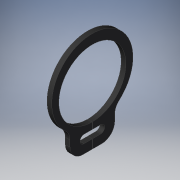
# Autodesk Inventor part: SL-STWS6
Saved by Autodesk Inventor 2019 (Build 230136000, 136)
## iProperties
Created: 2023-09-15
Part Number: SL-STWS6
Material: Generic
Catalog Web Link: www.cadenas.de
Description: SL-STWS, SH-STWS, SHD-STWS-(Precision cleaning) Retaining Rings - External, C-Type
Vendor: MISUMI
Document SubType Name: Modeling
Designer: psAdmin
Manufacturer: MISUMI
Mass: 0.00671227 g
Surface Area: 0.53562 cm^2
Volume: 0.00671227 cm^3
Density: 1 g/cm^3
Appearance: PSOLRGB-175-175-175
Category: PARTsolutions
Company: MISUMI
Title: SL-STWS6
Author: Cadenas PARTsolutions
Comments: (Precision cleaning) Retaining Rings - External, C-Type
PSOL_IDENT_0: {$CADENAS_DATA/23d-libs/misumi/metric/28_keys_magnets/sl_stws.prj},178 {VTYP=3D},{NB=SL-STWS6},{LINA=
PSOL_IDENT_1: SL-STWS6},{NN=SL-STWS, SH-STWS, SHD-STWS},{DATE=01.06.2023 05:14:51},{GEOMDATE=23.05.2023 07:22:17},
PSOL_IDENT_2: {VERSION=},{LINEID=40},{WBVAR=CM},{WBNUMERIC=}  {NB=SL-STWS6},{LINA=SL-STWS6},{KT=DUMMY},{PN=SL-STWS
PSOL_IDENT_3: 6},{TYPE=STWS},{TYPE0=SL-STWS},{MAT=2},{MATALG='1','Spring Steel','2','304 Stainless Steel-CSP'},{HA
PSOL_IDENT_4: RD=36~44HRC},{CM=SL},{NO=6},{DD3=5.5},{DD3TOL=+0.01/-0.01},{TT=0.40},{TTTOL=+0.04/-0.04},{BB=0.8},{A
PSOL_IDENT_5: A=2.0},{DD0=0.7},{DD4=12.0},{DD1=6},{DD2=5.7},{DD2TOL=+0.06/-0.06},{MM=0.45},{MMTOL=+0.10/0},{NN=1.5
PSOL_IDENT_6: },{H1=1.1},{A3=0.05},{A2=1.40},{A1=3.80},{R2=1.10},{R1=1.10}
NB: SL-STWS6
NN: 1.5
NT: (Precision cleaning) Retaining Rings - External, C-Type
NBSYN: $PN.
LINA: SL-STWS6
CATALOG: Misumi
PN: SL-STWS6
TYPE0: SL-STWS
MAT: 2
HARD: 36~44HRC
CM: Degreasing cleaning
NO: 6
DD3: 5.5
DD3TOL: +0.01/-0.01
TT: 0.4
TTTOL: +0.04/-0.04
BB: 0.8
AA: 2
DD0: 0.7
DD4: 12
DD1: 6
DD2: 5.7
DD2TOL: +0.06/-0.06
MM: 0.45
MMTOL: +0.10/0
SUPPLIER: MISUMI
ARTICLENO: SL-STWS6
BOMINFO: SL-STWS6
CREATOR: CADENAS GmbH
Autodesk Inventor part; units mm, degrees
sketch "Sketch_5" plane through (0, 0, 0) normal (1, 0, 0) x (0, 1, 0)
  arc A0 (-2.3939, -2.2747) -> (-2.3939, 2.2747) centre (0.2, 0) ccw
  arc A1 (-3.2209, 1.9) -> (-2.3939, 2.2747) centre (-3.2209, 3) ccw
  line L0 (-3.2209, 1.9) -> (-3.75, 1.9)
  arc A2 (-3.75, 1.9) -> (-4.85, 0.8) centre (-3.75, 0.8) ccw
  line L1 (-4.85, 0.8) -> (-4.85, 0.025)
  line L2 (-4.85, 0.025) -> (-4.1, 0.025)
  line L3 (-4.1, 0.025) -> (-4.1, 0.7)
  arc A3 (-3.4, 0.7) -> (-4.1, 0.7) centre (-3.75, 0.7) ccw
  line L4 (-3.4, 0.7) -> (-3.4, 0.025)
  line L5 (-3.4, 0.025) -> (-2.8499, 0.025)
  arc A4 (-2.8499, -0.025) -> (-2.8499, 0.025) centre (0, 0) ccw
  line L6 (-2.8499, -0.025) -> (-3.4, -0.025)
  line L7 (-3.4, -0.025) -> (-3.4, -0.7)
  arc A5 (-4.1, -0.7) -> (-3.4, -0.7) centre (-3.75, -0.7) ccw
  line L8 (-4.1, -0.7) -> (-4.1, -0.025)
  line L9 (-4.1, -0.025) -> (-4.85, -0.025)
  line L10 (-4.85, -0.025) -> (-4.85, -0.8)
  arc A6 (-4.85, -0.8) -> (-3.75, -1.9) centre (-3.75, -0.8) ccw
  line L11 (-3.75, -1.9) -> (-3.2209, -1.9)
  arc A7 (-2.3939, -2.2747) -> (-3.2209, -1.9) centre (-3.2209, -3) ccw
  constraints: 24 end point, 16 point on circle, 8 centre point
extrude "Extrusion1" add sketch "Sketch_5" along normal mid plane 0.4
ref_plane "1_XY" through (0, 0, 0) normal (1, 0, 0) x (0, 0, -1)
ref_plane "1_YZ" through (0, 0, 0) normal (0, 0, -1) x (0, 1, 0)
ref_plane "1_ZX" through (0, 0, 0) normal (0, 1, 0) x (1, 0, 0)
ref_plane "combination_module_XY" through (0.2, 0, 0) normal (1, 0, 0) x (0, 0, -1)
ref_plane "combination_module_YZ" through (0.2, 0, 0) normal (0, 0, -1) x (0, 1, 0)
ref_plane "combination_module_ZX" through (0.2, 0, 0) normal (0, 1, 0) x (1, 0, 0)
body "Solid1"
